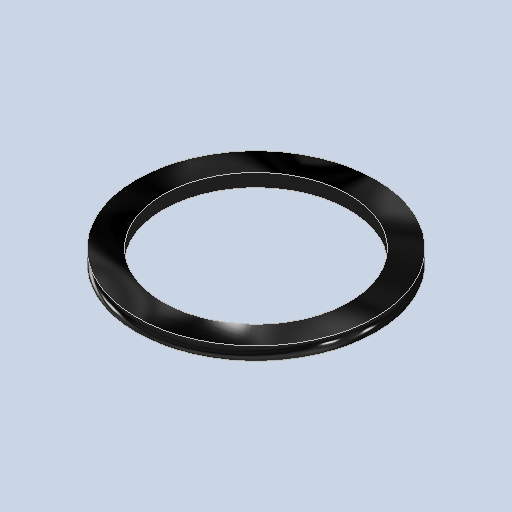
# Autodesk Inventor part: TorsOsc-2025-Cell-PCBGlue
Saved by Autodesk Inventor 2026 (Build 300175050, 175E)
## iProperties
Created: 2025-08-12
Part Number: TorsOsc-2025-Cell-PCBGlue
Material: Epoxy Resin
Document SubType Name: Modeling
Designer: schanen
Density: 1.14 g/cm^3
Appearance: Black
Author: schanen
Autodesk Inventor part; units mm, degrees
ref_plane "YZ Plane" through (0, 0, 0) normal (1, 0, 0) x (0, 1, 0)
ref_plane "XZ Plane" through (0, 0, 0) normal (0, 1, 0) x (-1, 0, 0)
ref_plane "XY Plane" through (0, 0, 0) normal (0, 0, 1) x (1, 0, 0)
sketch "Sketch1" plane through (0, 0, 0) normal (0, 0, 1) x (1, 0, 0)
  line L0 (-3.5, 0) -> (-3.5, 0.5)
  line L1 (-3.5, 0.5) -> (-4.5, 0.5)
  line L2 (-3.5, 0) -> (-4.5, 0)
  arc A0 (-4.5, 0) -> (-4.5, 0.5) centre (-4.5, 0.25) ccw
  line L3 (0, -0.1) -> (0, 0.6) projected
  point P0 (0, 0)
  dimension "d0" = 0.25
  dimension "d1" = 1
  dimension "d2" = 3.5
  dimension "d3" = 0.5
  constraints: 6 end point, 2 point on circle, 1 centre point, 1 horizontal, 1 horizontal alignment, 1 perpendicular, 1 vertical, 1 vertical alignment
  measures "d0" radius of A0
  measures "d1" distance of L0.start L2.end
  measures "d2" distance from line of point (0, 0) L0
  measures "d3" distance of L0.start L0.end
revolve "Revolution1" add sketch "Sketch1" angle 360 about axis through (0, -10, 0) along (0, 1, 0)
body "Solid1"
